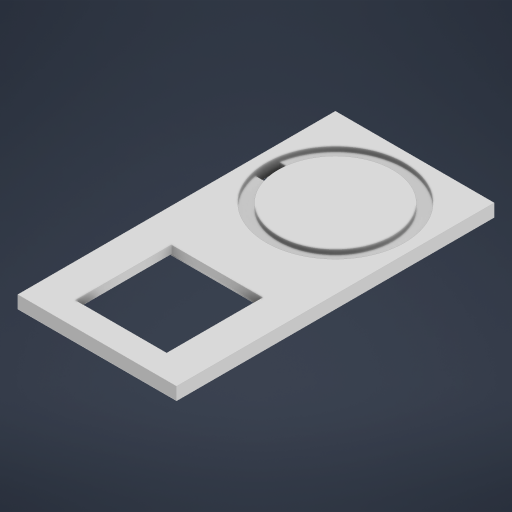
# Autodesk Inventor part: ViesCooleHouder
Saved by Autodesk Inventor 2023 (Build 270158000, 158)
## iProperties
Created: 2024-04-18
Part Number: ViesCooleHouder
Material: Generic
Document SubType Name: Modeling
Designer: warre
Density: 1 g/cm^3
Appearance: Default
Author: warre
Autodesk Inventor part; units mm, degrees
ref_plane "YZ Plane" through (0, 0, 0) normal (1, 0, 0) x (0, 1, 0)
ref_plane "XZ Plane" through (0, 0, 0) normal (0, 1, 0) x (-1, 0, 0)
ref_plane "XY Plane" through (0, 0, 0) normal (0, 0, 1) x (1, 0, 0)
sketch "Sketch1" plane through (0, 0, 0) normal (0, 1, 0) x (-1, 0, 0)
  line L0 (-50, 100) -> (50, 100)
  line L1 (50, 100) -> (50, -100)
  line L2 (50, -100) -> (-50, -100)
  line L3 (-50, -100) -> (-50, 100)
  line L4 (-50, 100) -> (50, -100) construction
  line L5 (50, 100) -> (-50, -100) construction
  circle A0 centre (0, -50) radius 43.5
  circle A1 centre (0, -50) radius 36
  line L6 (-28.75, 85) -> (28.75, 85)
  line L7 (28.75, 85) -> (28.75, 24.5)
  line L8 (28.75, 24.5) -> (-28.75, 24.5)
  line L9 (-28.75, 24.5) -> (-28.75, 85)
  line L10 (-28.75, 85) -> (28.75, 24.5) construction
  line L11 (28.75, 85) -> (-28.75, 24.5) construction
  point P0 (0, 0)
  point P1 (0, 54.75)
  dimension "d0" = 7.5
  dimension "d1" = 72
  dimension "d2" = 60.5
  dimension "d3" = 57.5
  dimension "d4" = 100
  dimension "d5" = 200
  dimension "d6" = 15
  dimension "d7" = 50
  constraints: 24 end point, 4 midpoint, 4 parallel, 2 centre point, 2 horizontal, 2 perpendicular, 2 vertical alignment, 1 coincident
  measures "d0" radial gap between concentric circles of A0 A1
  measures "d1" diameter of A1
  measures "d2" distance of L6.end L7.end
  measures "d3" distance between parallel lines of L9 L7
  measures "d4" distance between parallel lines of L3 L1
  measures "d5" distance of L2.end L0.start
  measures "d6" distance between parallel lines of L0 L6
  measures "d7" distance from line of L2 A0.centre
extrude "Extrusion1" add sketch "Sketch1" along normal blind 8
extrude "Extrusion2" add sketch "Sketch1" along normal blind 5 contours A0
sketch "Sketch2" plane through (0, 0, 0) normal (0, -1, 0) x (1, 0, 0)
  line L0 (50, -100) -> (-50, -100) projected
  line L1 (50, 100) -> (50, -100) projected
  line L2 (-50, 100) -> (50, 100) projected
  line L3 (-50, -100) -> (-50, 100) projected
  line L4 (28.75, 85) -> (-28.75, 85) projected
  line L5 (28.75, 24.5) -> (28.75, 85) projected
  line L6 (-28.75, 24.5) -> (28.75, 24.5) projected
  line L7 (-28.75, 85) -> (-28.75, 24.5) projected
  line L8 (-36.25, 22.25) -> (32.75, 22.25)
  line L9 (32.75, 22.25) -> (32.75, 87.25)
  line L10 (32.75, 87.25) -> (-36.25, 87.25)
  line L11 (-36.25, 87.25) -> (-36.25, 22.25)
  line L12 (-36.25, 22.25) -> (32.75, 87.25) construction
  line L13 (32.75, 22.25) -> (-36.25, 87.25) construction
  point P0 (0, 0)
  point P1 (-1.75, 54.75)
  dimension "d12" = 69
  dimension "d13" = 65
  dimension "d14" = 4
  dimension "d15" = 2.25
  constraints: 12 end point, 2 midpoint, 2 parallel, 1 horizontal, 1 perpendicular
  measures "d12" distance of L10.end L9.end
  measures "d13" distance of L9.end L8.end
  measures "d14" distance between parallel lines of L5 L9
  measures "d15" distance between parallel lines of L10 L4
extrude "Extrusion3" cut sketch "Sketch2" against normal blind 3 contours L11 L10 L9 L8
sketch "Sketch3" plane through (0, 5, -50) normal (0, 1, 0) x (1, 0, 0)
  circle A0 centre (0, 0) radius 36 projected
  circle A1 centre (0, 0) radius 43.5 projected
  circle A2 centre (0, 0) radius 43.5 projected
  circle A3 centre (0, 0) radius 36 projected
  circle A4 centre (0, 0) radius 36 projected
  line L0 (50, 50) -> (-50, 50) projected
  line L1 (-50, 50) -> (-50, -150) projected
  line L2 (-50, -150) -> (50, -150) projected
  line L3 (50, -150) -> (50, 50) projected
  line L4 (28.75, -135) -> (-28.75, -135) projected
  line L5 (-28.75, -135) -> (-28.75, -74.5) projected
  line L6 (-28.75, -74.5) -> (28.75, -74.5) projected
  line L7 (28.75, -74.5) -> (28.75, -135) projected
  circle A5 centre (0, 0) radius 43.5 projected
  line L8 (-35.2101, 7.5) -> (-42.8486, 7.5)
  line L9 (-42.8486, -7.5) -> (-35.2101, -7.5)
  point P0 (0, -50)
  point P1 (-39.0293, -7.5)
  point P2 (-35.2101, 7.5)
  point P3 (-42.8486, 7.5)
  dimension "d18" = 15
  constraints: 4 end point, 4 point on circle, 1 horizontal, 1 midpoint, 1 parallel, 1 vertical alignment
  measures "d18" distance from line of point (-39.029, -7.5) L8
extrude "Extrusion4" cut sketch "Sketch3" against normal through all contours A0 L9 A1 L8 picked at (-37.9902, -5.8388)
sketch "Sketch4" plane through (0, 0, 0) normal (0, -1, 0) x (1, 0, 0)
  arc A0 (-35.2101, -57.5) -> (-35.2101, -42.5) centre (0, -50) ccw projected
  arc A1 (-42.8486, -57.5) -> (-42.8486, -42.5) centre (0, -50) ccw projected
  line L0 (-30.5, -30) -> (30.5, -30)
  line L1 (30.5, -30) -> (30.5, -70)
  line L2 (30.5, -70) -> (-30.5, -70)
  line L3 (-30.5, -70) -> (-30.5, -30)
  line L4 (-30.5, -30) -> (30.5, -70) construction
  line L5 (30.5, -30) -> (-30.5, -70) construction
  point P0 (0, 0)
  point P1 (-30.5, -30.8754)
  point P2 (-30.5, -69.1246)
  point P3 (-29.9333, -70)
  point P4 (29.9333, -70)
  point P5 (30.5, -69.1246)
  point P6 (30.5, -30.8754)
  point P7 (29.9333, -30)
  point P8 (-29.9333, -30)
  dimension "d21" = 40
  dimension "d22" = 61
  constraints: 12 end point, 2 midpoint, 2 parallel, 1 horizontal, 1 perpendicular
  measures "d21" distance of L0.end L1.end
  measures "d22" distance of L1.end L2.end
extrude "Extrusion5" cut sketch "Sketch4" against normal blind 2 contours L3 A0 L0 L1 L2
body "Solid1"
